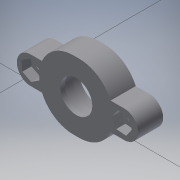
# Autodesk Inventor part: ппрофиль
Saved by Autodesk Inventor 2019 (Build 230136000, 136)
## iProperties
Created: 2022-06-29
Part Number: ппрофиль
Material: Типовые
Document SubType Name: Modeling
Designer: korsh
Density: 1 g/cm^3
Appearance: По умолчанию
Author: korsh
Autodesk Inventor part; units mm, degrees
ref_plane "YZ Plane" through (0, 0, 0) normal (1, 0, 0) x (0, 1, 0)
ref_plane "XZ Plane" through (0, 0, 0) normal (0, 1, 0) x (-1, 0, 0)
ref_plane "XY Plane" through (0, 0, 0) normal (0, 0, 1) x (1, 0, 0)
sketch "Эскиз1" plane through (0, 0, 0) normal (0, 0, 1) x (1, 0, 0)
  circle A0 centre (33.0944, 52) radius 10 projected
  circle A1 centre (53.0944, 52) radius 2 projected
  circle A2 centre (13.0944, 52) radius 2 projected
  line L0 (48.0944, 37) -> (18.0944, 37)
  line L1 (18.0944, 37) -> (18.0944, 67)
  line L2 (18.0944, 67) -> (48.0944, 67)
  line L3 (48.0944, 67) -> (48.0944, 37)
  line L4 (18.0944, 46) -> (7.0944, 46)
  line L5 (7.0944, 46) -> (7.0944, 58)
  line L6 (7.0944, 58) -> (18.0944, 58)
  line L7 (18.0944, 58) -> (18.0944, 46)
  line L8 (48.0944, 46) -> (60.0944, 46)
  line L9 (60.0944, 46) -> (60.0944, 58)
  line L10 (60.0944, 58) -> (48.0944, 58)
  line L11 (48.0944, 58) -> (48.0944, 46)
  point P0 (0, 0)
  dimension "d0" = 15
  dimension "d1" = 15
  dimension "d2" = 15
  dimension "d3" = 15
  dimension "d4" = 6
  dimension "d5" = 6
  dimension "d6" = 6
  dimension "d7" = 12
  dimension "d8" = 12
  constraints: 24 end point, 6 parallel, 3 horizontal, 3 perpendicular, 2 point on line
  measures "d0" distance from line of L1 A0.centre
  measures "d1" distance from line of L3 A0.centre
  measures "d2" distance from line of A0.centre L0
  measures "d3" distance from line of A0.centre L2
  measures "d4" distance from line of L4 A2.centre
  measures "d5" distance from line of A2.centre L5
  measures "d6" distance from line of L6 A2.centre
  measures "d7" distance between parallel lines of L10 L8
  measures "d8" distance between parallel lines of L9 L3
extrude "Выдавливание1" add sketch "Эскиз1" along normal blind 4
fillet "Сопряжение1" radius 15 4 edges at (18.0944, 37, 2) (18.0944, 67, 2) (48.0944, 37, 2) (48.0944, 67, 2)
fillet "Сопряжение2" radius 6 4 edges at (60.0944, 58, 2) (60.0944, 46, 2) (7.0944, 46, 2) (7.0944, 58, 2)
sketch "Эскиз2" plane through (0, 0, 4) normal (0, 0, 1) x (1, 0, 0)
  circle A0 centre (33.0944, 52) radius 10 projected
  circle A1 centre (33.0944, 52) radius 8.75
  circle A2 centre (33.0944, 52) radius 10 projected
  circle A3 centre (53.0944, 52) radius 2 projected
  circle A4 centre (13.0944, 52) radius 2 projected
  arc A5 (13.0944, 58) -> (13.0944, 46) centre (13.0944, 52) ccw projected
  line L0 (13.0944, 46) -> (18.0944, 46) projected
  arc A6 (18.0944, 46) -> (31.8421, 37) centre (31.8421, 52) ccw projected
  line L1 (31.8421, 37) -> (34.3467, 37) projected
  arc A7 (34.3467, 37) -> (48.0944, 46) centre (34.3467, 52) ccw projected
  line L2 (48.0944, 46) -> (54.0944, 46) projected
  arc A8 (54.0944, 46) -> (54.0944, 58) centre (54.0944, 52) ccw projected
  line L3 (54.0944, 58) -> (48.0944, 58) projected
  arc A9 (48.0944, 58) -> (34.3467, 67) centre (34.3467, 52) ccw projected
  line L4 (34.3467, 67) -> (31.8421, 67) projected
  arc A10 (31.8421, 67) -> (18.0944, 58) centre (31.8421, 52) ccw projected
  line L5 (18.0944, 58) -> (13.0944, 58) projected
  point P0 (0, 0)
  dimension "d13" = 17.5
  constraints: 1 centre point, 1 coincident
  measures "d13" diameter of A1
extrude "Выдавливание2" add sketch "Эскиз2" along normal blind 5 contours A0 | L5 A10 L4 A9 L3 A8 L2 A7 L1 A6 L0 A5
sketch "Эскиз3" plane through (0, 0, 9) normal (0, 0, 1) x (1, 0, 0)
  circle A0 centre (33.0944, 52) radius 8.75 projected
  circle A1 centre (13.0944, 52) radius 2 projected
  circle A2 centre (53.0944, 52) radius 2 projected
  arc A3 (13.0944, 58) -> (13.0944, 46) centre (13.0944, 52) ccw projected
  line L0 (13.0944, 46) -> (18.0944, 46) projected
  arc A4 (18.0944, 46) -> (31.8421, 37) centre (31.8421, 52) ccw projected
  line L1 (31.8421, 37) -> (34.3467, 37) projected
  arc A5 (34.3467, 37) -> (48.0944, 46) centre (34.3467, 52) ccw projected
  line L2 (48.0944, 46) -> (54.0944, 46) projected
  arc A6 (54.0944, 46) -> (54.0944, 58) centre (54.0944, 52) ccw projected
  line L3 (54.0944, 58) -> (48.0944, 58) projected
  arc A7 (48.0944, 58) -> (34.3467, 67) centre (34.3467, 52) ccw projected
  line L4 (34.3467, 67) -> (31.8421, 67) projected
  arc A8 (31.8421, 67) -> (18.0944, 58) centre (31.8421, 52) ccw projected
  line L5 (18.0944, 58) -> (13.0944, 58) projected
  circle A9 centre (33.0944, 52) radius 7
  point P0 (0, 0)
  dimension "d16" = 14
  constraints: 1 centre point, 1 coincident
  measures "d16" diameter of A9
extrude "Выдавливание3" add sketch "Эскиз3" along normal blind 2 contours A0 | L5 A8 L4 A7 L3 A6 L2 A5 L1 A4 L0 A3
sketch "Эскиз4" plane through (0, 0, 11) normal (0, 0, 1) x (1, 0, 0)
  circle A0 centre (13.0944, 52) radius 2 projected
  circle A1 centre (53.0944, 52) radius 2 projected
  line L0 (9.4717, 49.6281) -> (9.2289, 53.9514)
  line L1 (9.2289, 53.9514) -> (12.8516, 56.3233)
  line L2 (12.8516, 56.3233) -> (16.7171, 54.3719)
  line L3 (16.7171, 54.3719) -> (16.9599, 50.0486)
  line L4 (16.9599, 50.0486) -> (13.3372, 47.6767)
  line L5 (13.3372, 47.6767) -> (9.4717, 49.6281)
  line L6 (50.591, 48.4669) -> (48.7829, 52.4014)
  line L7 (48.7829, 52.4014) -> (51.2863, 55.9346)
  line L8 (51.2863, 55.9346) -> (55.5978, 55.5331)
  line L9 (55.5978, 55.5331) -> (57.4059, 51.5986)
  line L10 (57.4059, 51.5986) -> (54.9025, 48.0654)
  line L11 (54.9025, 48.0654) -> (50.591, 48.4669)
  point P0 (0, 0)
  dimension "d19" = 7.5
  dimension "d20" = 7.5
  constraints: 24 end point, 2 coincident, 26 other
  measures "d19" distance between parallel lines of L2 L5
  measures "d20" distance between parallel lines of L8 L11
extrude "Выдавливание4" cut sketch "Эскиз4" against normal blind 4
equation "\"d20\" = d19"
